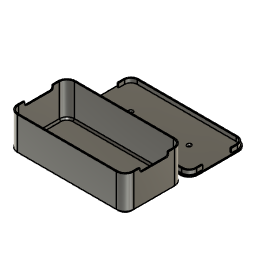
Cable Organizer (Autodesk Fusion 360 design; units mm, degrees)
Autodesk Fusion 360 part; units mm, degrees
note: some values were not read from the file. Set by a fixed rule: which face or edge a step refers to.
sketch "Case Sketch" plane through (0, 0, 0) normal (0, 0, 1) x (1, 0, 0) in component "Case Closure"
  line L0 (0, 0) -> (200, 0)
  line L1 (200, 0) -> (200, 100)
  line L2 (200, 100) -> (0, 100)
  line L3 (0, 100) -> (0, 0)
  dimension "d1" = 200
  dimension "d2" = 100
  constraint horizontal L0
  constraint vertical L1
  constraint horizontal L2
  constraint vertical L3
  constraint coincident L0.start L3.end
  measures "d1" distance of L0.start L0.end
  measures "d2" distance of L0.start L2.end
extrude "Extrude1" add sketch "Case Sketch" along normal blind 60 makes body 1 in component "Case Closure"
fillet "Fillet1" radius 15 4 edges at (200, 0, 30) (200, 100, 30) (0, 0, 30) (0, 100, 30) on bodies 1 in component "Case Closure"
chamfer "Chamfer1" distance 4 angle 45 1 faces at (128.3333, 33.3333, 0) on bodies 1 in component "Case Closure"
shell "Shell1" thickness 2 removed faces 1 at (128.3333, 33.3333, 60) on bodies 1 in component "Case Closure"
sketch "Holes Sketch" plane through (0, 0, 0) normal (-1, 0, 0) x (0, -1, 0) in component "Case Closure"
  line L0 (-85, 4) -> (-15, 4)
  line L1 (-15, 4) -> (-15, 60)
  line L2 (-15, 60) -> (-85, 60)
  line L3 (-85, 60) -> (-85, 4)
  line L4 (-50, 60) -> (-50, 4) construction
  line L5 (-29, 53) -> (-71, 53)
  line L6 (-74.5, 56.5) -> (-74.5, 60)
  line L7 (-74.5, 60) -> (-25.5, 60)
  line L8 (-25.5, 60) -> (-25.5, 56.5)
  line L9 (-25.5, 53) -> (-74.5, 60) construction
  line L10 (-74.5, 53) -> (-25.5, 60) construction
  arc A0 (-74.5, 56.5) -> (-71, 53) centre (-71, 56.5) ccw
  arc A1 (-29, 53) -> (-25.5, 56.5) centre (-29, 56.5) ccw
  point P0 (-50, 56.5)
  dimension "d32" = 49
  dimension "d33" = 7
  dimension "d34" = 3.5
  dimension "d35" = 3.5
  constraint midpoint L2 L4.start
  constraint midpoint L0 L4.end
  constraint horizontal L5
  constraint perpendicular L5 L6
  constraint parallel L5 L7
  constraint parallel L6 L8
  constraint coincident L9 P0
  constraint coincident L10 P0
  constraint coincident L4 P0
  constraint coincident L4.start L7
  constraint coincident L10.start L5
  constraint coincident L10.start L6
  constraint tangent L5 A0
  constraint tangent L6 A0
  constraint coincident L9.start L5
  constraint coincident L9.start L8
  constraint tangent L5 A1
  constraint tangent L8 A1
  measures "d32" distance of L6.end L7.end
  measures "d33" distance of L10.start L6.end
  measures "d34" radius of A0
  measures "d35" radius of A1
extrude "Extrude2" cut sketch "Holes Sketch" against normal up to surface (2 mm away) contours L2 L5 L6 L7 L8 A0 A1 bodies 1 in component "Case Closure"
ref_plane "WorkPlane1" through (100, 50, 30) normal (-1, 0, 0) x (0, -1, 0) in component "Case Closure"
mirror "Mirror1" about plane through (100, 50, 30) normal (-1, 0, 0) of "Extrude2" in component "Case Closure"
sketch "Case Lid Sketch" plane through (0, 0, 0) normal (0, 0, 1) x (1, 0, 0) in component "Case Lid"
  line L0 (0, 0) -> (200, 0)
  line L1 (200, 0) -> (200, 100)
  line L2 (200, 100) -> (0, 100)
  line L3 (0, 100) -> (0, 0)
  dimension "d23" = 200
  dimension "d24" = 100
  constraint horizontal L0
  constraint vertical L1
  constraint horizontal L2
  constraint vertical L3
  constraint coincident L0.start L3.end
  measures "d23" distance of L0.start L0.end
  measures "d24" distance of L0.start L2.end
extrude "Extrude1'" add sketch "Case Lid Sketch" along normal blind 2 separate body makes body 2 in component "Case Lid"
fillet "Fillet1'" radius 15 4 edges at (200, 0, 1) (200, 100, 1) (0, 100, 1) (0, 0, 1) on bodies 2 in component "Case Lid"
sketch "Case Lid Edge Sketch" plane through (0, 0, 2) normal (0, 0, 1) x (-1, 0, 0) in component "Case Lid"
  arc A0 (0, -15) -> (-15, 0) centre (-15, -15) ccw
  line L0 (-15, 0) -> (-185, 0)
  arc A1 (-185, 0) -> (-200, -15) centre (-185, -15) ccw
  line L1 (-200, -15) -> (-200, -85)
  arc A2 (-200, -85) -> (-185, -100) centre (-185, -85) ccw
  line L2 (-185, -100) -> (-15, -100)
  arc A3 (-15, -100) -> (0, -85) centre (-15, -85) ccw
  line L3 (0, -85) -> (0, -15)
  line L4 (-15, -2.1) -> (-185, -2.1)
  arc A4 (-185, -2.1) -> (-197.9, -15) centre (-185, -15) ccw
  line L5 (-197.9, -15) -> (-197.9, -85)
  arc A5 (-197.9, -85) -> (-185, -97.9) centre (-185, -85) ccw
  line L6 (-185, -97.9) -> (-15, -97.9)
  arc A6 (-15, -97.9) -> (-2.1, -85) centre (-15, -85) ccw
  line L7 (-2.1, -85) -> (-2.1, -15)
  arc A7 (-2.1, -15) -> (-15, -2.1) centre (-15, -15) ccw
  line L8 (-15, -4.1) -> (-185, -4.1)
  arc A8 (-185, -4.1) -> (-195.9, -15) centre (-185, -15) ccw
  line L9 (-195.9, -15) -> (-195.9, -85)
  arc A9 (-195.9, -85) -> (-185, -95.9) centre (-185, -85) ccw
  line L10 (-185, -95.9) -> (-15, -95.9)
  arc A10 (-15, -95.9) -> (-4.1, -85) centre (-15, -85) ccw
  line L11 (-4.1, -85) -> (-4.1, -15)
  arc A11 (-4.1, -15) -> (-15, -4.1) centre (-15, -15) ccw
  dimension "d48" = -4.1
extrude "Extrude2'" add sketch "Case Lid Edge Sketch" along normal blind 7 contours L4 A4 L5 A5 L6 A6 L7 A7 bodies 2 in component "Case Lid"
sketch "Case Lid Holes Sketch" plane through (197.9, 0, 0) normal (1, 0, 0) x (0, 1, 0) in component "Case Lid"
  line L0 (15, 2) -> (85, 2)
  line L1 (85, 2) -> (85, 9)
  line L2 (85, 9) -> (15, 9)
  line L3 (15, 9) -> (15, 2)
  line L4 (50, 9) -> (50, 2) construction
  line L5 (74.5, 2) -> (25.5, 2)
  line L6 (25.5, 2) -> (25.5, 9)
  line L7 (25.5, 9) -> (74.5, 9)
  line L8 (74.5, 9) -> (74.5, 2)
  line L9 (74.5, 2) -> (25.5, 9) construction
  line L10 (25.5, 2) -> (74.5, 9) construction
  point P0 (50, 5.5)
  dimension "d49" = 49
  dimension "d50" = 7
  constraint midpoint L2 L4.start
  constraint midpoint L0 L4.end
  constraint horizontal L5
  constraint perpendicular L5 L6
  constraint parallel L5 L7
  constraint parallel L6 L8
  constraint coincident L9 P0
  constraint coincident L10 P0
  constraint midpoint L4 P0
  measures "d49" distance of L6.end L7.end
  measures "d50" distance of L5.end L6.end
extrude "Extrude4" cut sketch "Case Lid Holes Sketch" against normal up to surface (2 mm away) contours L0 L2 L5 L6 L7 L8 bodies 2 in component "Case Lid"
ref_plane "WorkPlane1" through (100, 50, 5.5) normal (1, 0, 0) x (0, 1, 0)
mirror "Mirror2" about plane through (100, 50, 5.5) normal (1, 0, 0) of "Extrude4" in component "Case Lid"
sketch "Case Lid Screw Holes Sketch" plane through (0, 0, 2) normal (0, 0, 1) x (-1, 0, 0) in component "Case Lid"
  line L0 (-2.1, -74.5) -> (-2.1, -85)
  arc A0 (-15, -97.9) -> (-2.1, -85) centre (-15, -85) ccw
  line L1 (-15, -97.9) -> (-185, -97.9)
  arc A1 (-197.9, -85) -> (-185, -97.9) centre (-185, -85) ccw
  line L2 (-197.9, -85) -> (-197.9, -74.5)
  line L3 (-197.9, -74.5) -> (-195.9, -74.5)
  line L4 (-195.9, -74.5) -> (-195.9, -85)
  arc A2 (-195.9, -85) -> (-185, -95.9) centre (-185, -85) ccw
  line L5 (-185, -95.9) -> (-15, -95.9)
  arc A3 (-15, -95.9) -> (-4.1, -85) centre (-15, -85) ccw
  line L6 (-4.1, -85) -> (-4.1, -74.5)
  line L7 (-4.1, -74.5) -> (-2.1, -74.5)
  arc A4 (0, -15) -> (-15, 0) centre (-15, -15) ccw
  line L8 (-15, 0) -> (-185, 0)
  arc A5 (-185, 0) -> (-200, -15) centre (-185, -15) ccw
  line L9 (-200, -15) -> (-200, -85)
  arc A6 (-200, -85) -> (-185, -100) centre (-185, -85) ccw
  line L10 (-185, -100) -> (-15, -100)
  arc A7 (-15, -100) -> (0, -85) centre (-15, -85) ccw
  line L11 (0, -85) -> (0, -15)
  line L12 (-2.1, -25.5) -> (-4.1, -25.5)
  line L13 (-4.1, -25.5) -> (-4.1, -15)
  arc A8 (-4.1, -15) -> (-15, -4.1) centre (-15, -15) ccw
  line L14 (-15, -4.1) -> (-185, -4.1)
  arc A9 (-185, -4.1) -> (-195.9, -15) centre (-185, -15) ccw
  line L15 (-195.9, -15) -> (-195.9, -25.5)
  line L16 (-195.9, -25.5) -> (-197.9, -25.5)
  line L17 (-197.9, -25.5) -> (-197.9, -15)
  arc A10 (-185, -2.1) -> (-197.9, -15) centre (-185, -15) ccw
  line L18 (-185, -2.1) -> (-15, -2.1)
  arc A11 (-2.1, -15) -> (-15, -2.1) centre (-15, -15) ccw
  line L19 (-2.1, -15) -> (-2.1, -25.5)
  circle A12 centre (-50, -50) radius 1.7
  circle A13 centre (-150, -50) radius 1.7
  dimension "d56" = 3.4
  dimension "d57" = 50
  dimension "d60" = 3.4
  dimension "d61" = 50
  measures "d56" diameter of A12
  measures "d57" distance of L11 A12.centre
  measures "d60" diameter of A13
  measures "d61" distance of L9 A13.centre
extrude "Extrude5" cut sketch "Case Lid Screw Holes Sketch" against normal up to surface (2 mm away) contours A12 | A13 bodies 2 in component "Case Lid"
chamfer "Chamfer1'" distance 2 angle 45 2 edges at (151.585, 49.3853, 2) (51.585, 49.3853, 2) on bodies 2 in component "Case Lid"
component "Case Closure" placed x (1, 0, 0) y (0, 1, 0) z (0, 0, 1) at (0, 0, 0)
component "Case Lid" placed x (1, 0, 0) y (0, 1, 0) z (0, 0, 1) at (0, 0, 0)
equation "d1 = CaseWidth"
equation "d2 = CaseDepth"
equation "d3 = CaseHeight"
equation "d6 = FilletSize"
equation "FilletSize = 15 mm"
equation "d8 = ChamferSize"
equation "ChamferSize = 4 mm"
equation "CaseThickness = 2 mm"
equation "d11 = CaseThickness"
equation "HolesSize = 7 mm"
equation "d23 = CaseWidth"
equation "d24 = CaseDepth"
equation "CaseWidth = 200 mm"
equation "CaseDepth = 100 mm"
equation "CaseHeight = 60 mm"
equation "d28 = CaseThickness"
equation "d31 = FilletSize"
equation "d32 = HolesSize * CablesCount"
equation "d33 = HolesSize"
equation "d34 = HolesSize / 2"
equation "d35 = HolesSize / 2"
equation "d38 = HolesSize"
equation "JoinTolerance = 0.1 mm"
equation "d47 = -CaseThickness - JoinTolerance"
equation "d48 = -JoinTolerance - CaseThickness * 2"
equation "d49 = HolesSize * CablesCount"
equation "d50 = HolesSize"
equation "CablesCount = 7"
equation "d56 = ScrewSize"
equation "d57 = CaseWidth / 4"
equation "ScrewSize = 3.4 mm"
equation "d60 = ScrewSize"
equation "d61 = CaseWidth / 4"
